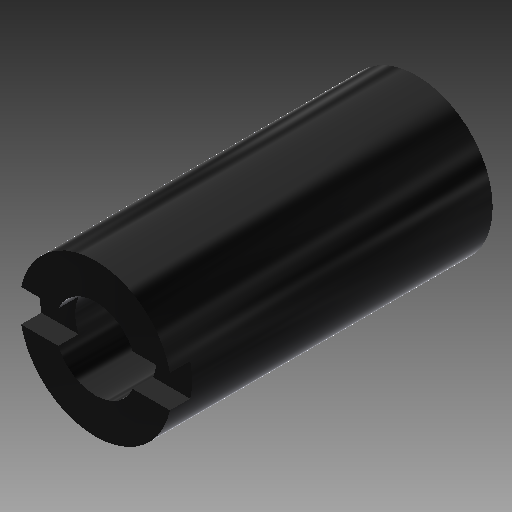
# Autodesk Inventor part: 308-10
Saved by Autodesk Inventor 2019 (Build 230136000, 136)
## iProperties
Company: Autodesk Inc.
Created: 2012-01-24
Part Number: 308-10
Material: PC/ABS Plastic
Document SubType Name: Modeling
Designer: Autodesk Inc.
Mass: 0.138833 g
Surface Area: 6.77865 cm^2
Volume: 0.388591 cm^3
Density: 0.357273 g/cm^3
Appearance: Smooth - Black
Author: Inventor
Autodesk Inventor part; units mm, degrees
ref_plane "YZ Plane" through (0, 0, 0) normal (1, 0, 0) x (0, 1, 0)
ref_plane "XZ Plane" through (0, 0, 0) normal (0, 1, 0) x (-1, 0, 0)
ref_plane "XY Plane" through (0, 0, 0) normal (0, 0, 1) x (1, 0, 0)
sketch "Sketch1" plane through (0, 0, 0) normal (0, 0, 1) x (1, 0, 0)
  circle A0 centre (0, 0) radius 3.75
  dimension "d0" = 7.5
  constraints: 1 centre point, 1 coincident
  measures "d0" diameter of A0
extrude "Extrusion1" add sketch "Sketch1" along normal blind 15.8
sketch "Sketch2" plane through (0, 0, 0) normal (0, 0, -1) x (-1, 0, 0)
  circle A0 centre (0, 0) radius 3.75 projected
  circle A1 centre (0, 0) radius 3.25
  dimension "d3" = 6.5
  constraints: 1 centre point, 1 coincident
  measures "d3" diameter of A1
extrude "Extrusion2" cut sketch "Sketch2" against normal blind 3 contours A1
hole "Hole1" at (0, 0, 3) direction (0, 0, 1) diameter 4.917 depth 6.75 thread size "M6x1" class "6H" standard "ANSI Metric M Profile"
hole "Hole2" at (0, 0, 15.8) direction (0, 0, -1) diameter 4 end through all
sketch "Sketch3" plane through (0, 0, 0) normal (1, 0, 0) x (0, 1, 0)
  line L0 (-2, 15.8) -> (2, 15.8) projected
  line L1 (0.8, 15.8) -> (-0.8, 15.8)
  line L2 (-0.8, 15.8) -> (-0.8, 14.8)
  line L3 (-0.8, 14.8) -> (0.8, 14.8)
  line L4 (0.8, 14.8) -> (0.8, 15.8)
  point P0 (0, 0)
  point P1 (0, 15.8)
  dimension "d26" = 1.6
  dimension "d27" = 1
  constraints: 8 end point, 2 midpoint, 2 parallel, 1 horizontal, 1 perpendicular
  measures "d26" distance of L3.end L2.end
  measures "d27" distance of L2.end L1.end
extrude "Extrusion3" cut sketch "Sketch3" along normal through all both and the other way through all
body "Solid1"
